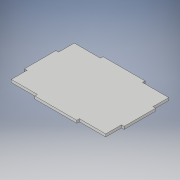
# Autodesk Inventor part: top
Saved by Autodesk Inventor 2019 (Build 230136000, 136)
## iProperties
Created: 2018-09-07
Part Number: top
Material: Generic
Document SubType Name: Modeling
Designer: mspet
Density: 1 g/cm^3
Appearance: Default
Author: mspet
Autodesk Inventor part; units mm, degrees
ref_plane "YZ Plane" through (0, 0, 0) normal (1, 0, 0) x (0, 1, 0)
ref_plane "XZ Plane" through (0, 0, 0) normal (0, 1, 0) x (-1, 0, 0)
ref_plane "XY Plane" through (0, 0, 0) normal (0, 0, 1) x (1, 0, 0)
sketch "Sketch1" plane through (0, 0, 0) normal (0, 1, 0) x (-1, 0, 0)
  line L0 (0, 0) -> (114.3, 0)
  line L1 (114.3, 0) -> (114.3, -76.2)
  line L2 (114.3, -76.2) -> (0, -76.2)
  line L3 (0, -76.2) -> (0, 0)
  dimension "d0" = 114.3
  dimension "d1" = 76.2
  constraints: 8 end point, 2 parallel, 1 horizontal, 1 perpendicular
  measures "d0" distance of L1.end L2.end
  measures "d1" distance of L0.end L1.end
extrude "Extrusion1" add sketch "Sketch1" along normal blind 3.175
sketch "Sketch2" plane through (0, 3.175, 0) normal (0, 1, 0) x (1, 0, 0)
  line L0 (-82.55, 0) -> (-31.75, 0)
  line L1 (-31.75, 0) -> (-31.75, -3.175)
  line L2 (-31.75, -3.175) -> (-82.55, -3.175)
  line L3 (-82.55, -3.175) -> (-82.55, 0)
  line L4 (-114.3, 0) -> (0, 0) projected
  line L5 (-114.3, 76.2) -> (-114.3, 0) projected
  line L6 (-114.3, 38.1) -> (-60.6343, 38.1) construction
  line L7 (-82.55, 76.2) -> (-31.75, 76.2)
  line L8 (-31.75, 76.2) -> (-31.75, 79.375)
  line L9 (-31.75, 79.375) -> (-82.55, 79.375)
  line L10 (-82.55, 79.375) -> (-82.55, 76.2)
  line L11 (-114.3, 76.2) -> (0, 76.2)
  line L12 (-114.3, 19.05) -> (-117.475, 19.05)
  line L13 (-117.475, 19.05) -> (-117.475, 57.15)
  line L14 (-117.475, 57.15) -> (-114.3, 57.15)
  line L15 (-114.3, 57.15) -> (-114.3, 19.05)
  line L16 (0, 76.2) -> (-114.3, 76.2) projected
  line L17 (-57.15, 76.2) -> (-57.15, 50.0024) construction
  line L18 (0, 76.2) -> (0, 0)
  line L19 (0, 38.1) -> (-53.6657, 38.1) construction
  line L20 (0, 19.05) -> (3.175, 19.05)
  line L21 (3.175, 19.05) -> (3.175, 57.15)
  line L22 (3.175, 57.15) -> (0, 57.15)
  line L23 (0, 57.15) -> (0, 19.05)
  dimension "d4" = 50.8
  dimension "d5" = 3.175
  dimension "d6" = 0
  dimension "d7" = 31.75
  dimension "d8" = 38.1
  dimension "d9" = 3.175
  dimension "d10" = 19.05
  constraints: 42 end point, 11 symmetric about line, 4 parallel, 3 horizontal, 2 midpoint, 2 perpendicular, 2 point on line, 1 vertical
  measures "d4" distance of L1.end L2.end
  measures "d5" distance of L0.end L1.end
  measures "d6" distance between parallel lines of L4 L0
  measures "d7" distance between parallel lines of L3 L5
  measures "d8" distance of L12.end L13.end
  measures "d9" distance of L12.start L12.end
  measures "d10" distance between parallel lines of L4 L12
extrude "Extrusion2" add sketch "Sketch2" against normal blind 3.175 contours L0 L1 L2 L3 | L12 L13 L14 L5 | L18 L22 L21 L20 | L10 L9 L8 L7
body "Solid1"
